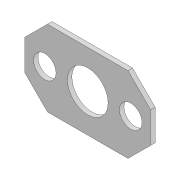
# Autodesk Inventor part: SlipersLåda 211018004
Saved by Autodesk Inventor 2020 (Build 240168000, 168)
## iProperties
Created: 2021-10-18
Part Number: SlipersLåda 211018004
Material: Generic
Document SubType Name: Modeling
Designer: dicpet001
Density: 1 g/cm^3
Appearance: Default
Author: dicpet001
Autodesk Inventor part; units mm, degrees
ref_plane "YZ Plane" through (0, 0, 0) normal (1, 0, 0) x (0, 1, 0)
ref_plane "XZ Plane" through (0, 0, 0) normal (0, 1, 0) x (-1, 0, 0)
ref_plane "XY Plane" through (0, 0, 0) normal (0, 0, 1) x (1, 0, 0)
sketch "Sketch1" plane through (0, 0, 0) normal (0, 0, 1) x (1, 0, 0)
  line L0 (0, 117.6) -> (0, -117.6) projected
  line L1 (-194.6, 0) -> (194.6, 0) projected
  line L2 (-89, 84) -> (89, 84)
  line L3 (139, 34) -> (139, -34)
  line L4 (89, -84) -> (-89, -84)
  line L5 (-139, -34) -> (-139, 34)
  circle A0 centre (-95, 0) radius 25
  circle A1 centre (95, 0) radius 25
  circle A2 centre (0, 0) radius 45
  line L6 (-89, 84) -> (-139, 34)
  line L7 (89, 84) -> (139, 34)
  line L8 (139, -34) -> (89, -84)
  line L9 (-89, -84) -> (-139, -34)
  point P0 (-139, 84)
  point P1 (139, 84)
  point P2 (-139, -84)
  point P3 (139, -84)
  dimension "d0" = 278
  dimension "d1" = 168
  dimension "d8" = 50
  dimension "d9" = 190
  dimension "d10" = 95
  dimension "d11" = 90
  dimension "d12" = 50
  dimension "d13" = 50
  dimension "d14" = 50
  dimension "d15" = 50
  dimension "d16" = 50
  dimension "d17" = 50
  dimension "d18" = 50
  dimension "d19" = 50
  constraints: 16 end point, 10 point on line, 3 centre point, 2 parallel, 1 coincident, 1 equal radius, 1 horizontal, 1 perpendicular, 2 other
  measures "d0" distance between parallel lines of L3 L5
  measures "d1" distance between parallel lines of L2 L4
  measures "d8" diameter of A0
  measures "d9" distance of A1.centre A0.centre
  measures "d10" distance from line of L0 A0.centre
  measures "d11" diameter of A2
  measures "d12" distance of L2.start point (-139, 84)
  measures "d13" distance of L5.end point (-139, 84)
  measures "d14" distance of L2.end point (139, 84)
  measures "d15" distance of L3.start point (139, 84)
  measures "d16" distance of L3.end point (139, -84)
  measures "d17" distance of L4.start point (139, -84)
  measures "d18" distance of L4.end point (-139, -84)
  measures "d19" distance of L5.start point (-139, -84)
extrude "Extrusion2" add sketch "Sketch1" against normal blind 10 contours L2 L7 L3 L1 A1 A2 L0 | L0 A2 L1 A0 L5 L6 L2 | L1 A1 L3 L8 L4 L0 A2 | A2 L0 L4 L9 L5 L1 A0
equation "\"d13\" = d12"
equation "\"d14\" = d12"
equation "\"d15\" = d14"
equation "\"d16\" = d12"
equation "\"d17\" = d16"
equation "\"d18\" = d12"
equation "\"d19\" = d18"
body "Solid2"
